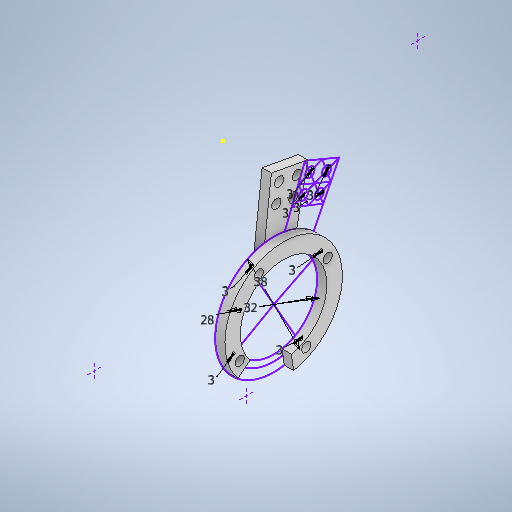
# Autodesk Inventor part: motor_mound
Saved by Autodesk Inventor 2025 (Build 290162000, 162)
## iProperties
Created: 2025-12-07
Part Number: motor_mound
Material: Типовые
Document SubType Name: Modeling
Designer: Admin
Density: 1 g/cm^3
Appearance: По умолчанию
Author: Admin
Autodesk Inventor part; units mm, degrees
ref_plane "YZ Plane" through (0, 0, 0) normal (1, 0, 0) x (0, 1, 0)
ref_plane "XZ Plane" through (0, 0, 0) normal (0, 1, 0) x (-1, 0, 0)
ref_plane "XY Plane" through (0, 0, 0) normal (0, 0, 1) x (1, 0, 0)
sketch "Эскиз1" plane through (0, 0, 0) normal (1, 0, 0) x (0, 1, 0)
  circle A0 centre (-54.1058, -16.5076) radius 16
  circle A1 centre (-54.1058, -16.5076) radius 14
  circle A2 centre (-54.1058, -16.5076) radius 19
  line L0 (-54.1058, -16.5076) -> (-62.8101, 0.3813)
  line L1 (-54.1058, -16.5076) -> (-45.4015, -33.3965)
  line L2 (-54.1058, -16.5076) -> (-70.9947, -25.2119)
  line L3 (-54.1058, -16.5076) -> (-37.6871, -6.9458)
  line L4 (-67.8834, -18.9928) -> (-72.8305, -19.73)
  line L5 (-62.9482, -5.6535) -> (-66.048, -1.7298)
  line L6 (-40.6156, -12.7639) -> (-16.8789, -15.5395)
  line L7 (-16.8789, -15.5395) -> (-19.0698, -27.3017)
  line L8 (-19.0698, -27.3017) -> (-41.5699, -22.7407)
  line L9 (-28.383, -14.1943) -> (-30.5675, -24.971)
  line L10 (-28.383, -14.1943) -> (-19.0698, -27.3017)
  line L11 (-30.5675, -24.971) -> (-16.8789, -15.5395)
  line L12 (-23.9604, -20.4186) -> (-22.9207, -14.833)
  line L13 (-22.9207, -14.833) -> (-29.4202, -19.3112)
  line L14 (-22.9207, -14.833) -> (-17.9743, -21.4206)
  line L15 (-23.9604, -20.4186) -> (-24.9531, -26.1091)
  line L16 (-17.9743, -21.4206) -> (-24.9429, -26.0503)
  line L17 (-29.4202, -19.3112) -> (-24.9429, -26.0503)
  circle A3 centre (-61.4358, -2.2854) radius 1.5
  circle A4 centre (-68.328, -23.8376) radius 1.5
  circle A5 centre (-46.7758, -30.7298) radius 1.5
  circle A6 centre (-40.2796, -8.4556) radius 1.5
  circle A7 centre (-26.2831, -17.1497) radius 1.5
  circle A8 centre (-20.5111, -18.0421) radius 1.5
  circle A9 centre (-21.5572, -23.8009) radius 1.5
  circle A10 centre (-27.201, -22.6514) radius 1.5
  point P0 (-6.6177, -23.1834)
  point P1 (-76.739, -12.454)
  point P2 (39.1344, -10.1827)
  point P3 (-35.3653, -13.3778)
  point P4 (-36.5442, -23.7594)
  dimension "d0" = 32
  dimension "d2" = 28
  dimension "d3" = 38
  dimension "d7" = 3
  dimension "d8" = 3
  dimension "d9" = 3
  dimension "d10" = 3
  dimension "d11" = 3
  dimension "d12" = 3
  dimension "d13" = 3
  dimension "d15" = 3
  constraints: 36 end point, 20 point on line, 14 point on circle, 11 centre point, 3 perpendicular, 2 coincident, 1 midpoint, 1 parallel
  measures "d0" diameter of A0
  measures "d2" diameter of A1
  measures "d3" diameter of A2
  measures "d7" diameter of A3
  measures "d8" diameter of A4
  measures "d9" diameter of A5
  measures "d10" diameter of A6
  measures "d11" diameter of A7
  measures "d12" diameter of A8
  measures "d13" diameter of A9
  measures "d15" diameter of A10
extrude "Выдавливание1" add sketch "Эскиз1" along normal blind 6 contours A0 L8 A1 L6 | A0 L6 A2 L8 | L6 A1 L3 A6 A0 | A0 A6 L3 A2 L6 | L8 A2 L1 A5 A0 | A0 A5 L1 A1 L8 | L3 A1 L0 A3 A0 A6 | L3 A6 A0 A3 L0 A2 | A5 A0 A4 L2 A1 L1 | A2 L2 A4 A0 A5 L1 | A1 L5 A0 A3 L0 | L0 A3 A0 L5 A2 | A2 L4 A0 A4 L2 | L2 A4 A0 L4 A1
extrude "Выдавливание2" add sketch "Эскиз1" along normal blind 3 contours L6 L9 L8 A2 | L10 A7 L13 L9 | L6 L13 A7 L10 | L11 A10 L17 L15 L8 | L9 L17 A10 L11 | L14 A8 L11 L12 | L12 L10 A7 L13 | L6 L11 A8 L14 | L13 A7 L10 L11 A10 L17 | L15 L16 A9 L10 L8 | L7 L14 A8 L11 | L11 A8 L14 L16 A9 L10 | L15 L17 A10 L11 | L10 A9 L16 L15 | L10 A9 L16 L7
extrude "Выдавливание3" cut sketch "Эскиз1" along normal blind 3 contours L6 A1 L3 A6 A0 | A0 A6 L3 A2 L6 | L8 A2 L1 A5 A0 | A0 A5 L1 A1 L8 | L3 A1 L0 A3 A0 A6 | L3 A6 A0 A3 L0 A2 | A5 A0 A4 L2 A1 L1 | A2 L2 A4 A0 A5 L1 | A1 L5 A0 A3 L0 | L0 A3 A0 L5 A2 | A2 L4 A0 A4 L2 | L2 A4 A0 L4 A1
sketch "Эскиз3" plane through (3, 0, 0) normal (-1, 0, 0) x (0, 0, 1)
  line L0 (-32.3349, -33.8419) -> (-22.1169, -29.7797)
  line L1 (-26.451, -18.878) -> (-17.9696, -40.2117)
  line L2 (-26.8452, -44.8668) -> (-37.4977, -23.4738)
  line L3 (-34.7862, -28.919) -> (-27.4833, -31.9131)
  line L4 (-27.4833, -31.9131) -> (-24.288, -24.4799)
  line L5 (-29.5408, -26.736) -> (-24.2332, -24.4564)
  line L6 (-37.4977, -23.4738) -> (-26.451, -18.878)
  line L7 (-31.9743, -21.1759) -> (-24.288, -24.4799)
  line L8 (-34.7862, -28.919) -> (-31.9743, -21.1759)
  line L9 (-22.1169, -29.7797) -> (-37.4977, -23.4738)
  line L10 (-32.3349, -33.8419) -> (-26.451, -18.878)
  line L11 (-29.5408, -26.736) -> (-34.7862, -28.919)
  line L12 (-16.3356, -54.116) -> (-33.3178, -45.5953)
  line L13 (-16.3356, -54.116) -> (-6.9524, -37.5946)
  line L14 (-20.5901, -67.4538) -> (-22.1809, -72.1945)
  line L15 (-16.3356, -54.116) -> (-25.7187, -70.6374)
  line L16 (-16.3356, -54.116) -> (0.1858, -63.4991)
  circle A0 centre (-16.3356, -54.116) radius 14
  circle A1 centre (-16.3356, -54.116) radius 16
  circle A2 centre (-16.3356, -54.116) radius 19
  line L17 (-6.7225, -64.2939) -> (-3.4007, -68.0332)
  circle A3 centre (-24.2372, -68.0287) radius 1.5
  circle A4 centre (-2.4228, -62.0176) radius 1.5
  circle A5 centre (-8.434, -40.2032) radius 1.5
  circle A6 centre (-30.6364, -46.9407) radius 1.5
  circle A7 centre (-31.0082, -30.4679) radius 1.5
  circle A8 centre (-33.4164, -25.147) radius 1.5
  circle A9 centre (-28.0225, -22.8746) radius 1.5
  circle A10 centre (-25.8996, -28.2288) radius 1.5
  point P0 (0, 0)
  point P1 (-7.3565, -75.2836)
  point P2 (-62.9166, -3.4682)
  point P3 (41.7851, -43.7086)
  point P4 (-32.7147, -46.9037)
  point P5 (-33.8935, -57.2853)
  dimension "d22" = 32
  dimension "d23" = 28
  dimension "d24" = 38
  dimension "d25" = 3
  dimension "d26" = 3
  dimension "d27" = 3
  dimension "d28" = 3
  dimension "d29" = 3
  dimension "d30" = 3
  dimension "d31" = 3
  dimension "d32" = 3
  constraints: 36 end point, 20 point on line, 14 point on circle, 11 centre point, 3 perpendicular, 2 coincident, 1 midpoint, 1 parallel
  measures "d22" diameter of A1
  measures "d23" diameter of A0
  measures "d24" diameter of A2
  measures "d25" diameter of A3
  measures "d26" diameter of A4
  measures "d27" diameter of A5
  measures "d28" diameter of A6
  measures "d29" diameter of A7
  measures "d30" diameter of A8
  measures "d31" diameter of A9
  measures "d32" diameter of A10
